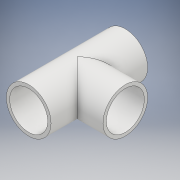
# Autodesk Inventor part: Piping_Tee_1.25in
Saved by Autodesk Inventor 2018 (Build 220112000, 112)
## iProperties
Created: 2018-10-21
Part Number: Piping_Tee_1.25in
Material: PVC-Piping
Document SubType Name: Modeling
Designer: Bradley
Density: 1.4 g/cm^3
Appearance: Smooth - White
Author: Bradley
Autodesk Inventor part; units mm, degrees
ref_plane "XZ Plane" through (0, 0, 0) normal (0, 1, 0) x (-1, 0, 0)
ref_plane "XY Plane" through (0, 0, 0) normal (0, 0, 1) x (1, 0, 0)
sketch "Sketch1" plane through (0, 0, 0) normal (0, 1, 0) x (-1, 0, 0)
  circle A0 centre (0, 0) radius 21.209
  circle A1 centre (0, 0) radius 24.892
  dimension "d0" = 42.418
  dimension "d1" = 49.784
  constraints: 2 centre point, 2 coincident
  measures "d0" diameter of A0
  measures "d1" diameter of A1
extrude "Extrusion1" add sketch "Sketch1" along normal mid plane 107.696
sketch "Sketch4" plane through (0, 0, 0) normal (0, 1, 0) x (-1, 0, 0)
  circle A0 centre (0, 0) radius 17.526
  circle A1 centre (0, 0) radius 21.209 projected
  circle A2 centre (0, 0) radius 24.892 projected
  dimension "d9" = 35.052
  constraints: 1 centre point, 1 coincident
  measures "d9" diameter of A0
extrude "Extrusion4" add sketch "Sketch4" along normal mid plane 44.45 contours A1
ref_plane "Work Plane1" through (53.848, 0, 0) normal (1, 0, 0) x (0, 1, 0)
sketch "Sketch2" plane through (53.848, 0, 0) normal (1, 0, 0) x (0, 1, 0)
  line L0 (-53.848, 24.892) -> (-53.848, -24.892) projected
  line L1 (53.848, -24.892) -> (53.848, 24.892) projected
  circle A0 centre (0, 0) radius 24.892
  line L2 (-53.848, 24.892) -> (53.848, 24.892) projected
  constraints: 1 centre point, 1 coincident, 1 tangent
extrude "Extrusion2" add sketch "Sketch2" against normal up to next
sketch "Sketch3" plane through (53.848, 0, 0) normal (1, 0, 0) x (0, 0, -1)
  line L0 (-21.209, -53.848) -> (-21.209, -22.225) projected
  circle A0 centre (0, 0) radius 21.209
  constraints: 1 centre point, 1 coincident, 1 tangent
extrude "Extrusion3" cut sketch "Sketch3" against normal blind 31.623
sketch "Sketch5" plane through (22.225, 0, 0) normal (1, 0, 0) x (0, 0, -1)
  line L0 (-17.526, -22.225) -> (-17.526, 22.225) projected
  circle A0 centre (0, 0) radius 17.526
  constraints: 1 centre point, 1 coincident, 1 tangent
extrude "Extrusion5" cut sketch "Sketch5" against normal up to next
body "Solid1"
